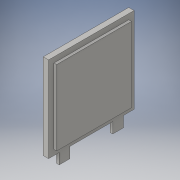
# Autodesk Inventor part: top
Saved by Autodesk Inventor 2016 (Build 200138000, 138)
## iProperties
Created: 2016-08-07
Part Number: top
Material: Generic
Document SubType Name: Modeling
Designer: Jorian Brusind
Density: 1 g/cm^3
Appearance: Default
Author: Jorian Brusind
Autodesk Inventor part; units mm, degrees
ref_plane "YZ Plane" through (0, 0, 0) normal (1, 0, 0) x (0, 1, 0)
ref_plane "XZ Plane" through (0, 0, 0) normal (0, 1, 0) x (-1, 0, 0)
ref_plane "XY Plane" through (0, 0, 0) normal (0, 0, 1) x (1, 0, 0)
sketch "Sketch1" plane through (0, 0, 0) normal (0, 1, 0) x (-1, 0, 0)
  line L0 (0, 0) -> (6.35, 0)
  line L1 (6.35, 0) -> (6.35, -101.6)
  line L2 (6.35, -101.6) -> (0, -101.6)
  line L3 (0, -101.6) -> (0, 0)
  dimension "d0" = 6.35
  dimension "d1" = 101.6
  constraints: 8 end point, 2 parallel, 1 horizontal, 1 perpendicular
  measures "d0" distance of L1.end L2.end
  measures "d1" distance of L0.end L1.end
extrude "Extrusion1" add sketch "Sketch1" along normal blind 101.6
sketch "Sketch2" plane through (0, 0, 0) normal (0, -1, 0) x (1, 0, 0)
  line L0 (0, 0) -> (0, -25.4)
  line L1 (0, 0) -> (0, -101.6) projected
  line L2 (0, -101.6) -> (0, -76.2)
  line L3 (0, -25.4) -> (-3.175, -25.4)
  line L4 (-3.175, -25.4) -> (-3.175, -12.7)
  line L5 (-3.175, -12.7) -> (0, -12.7)
  line L6 (0, -12.7) -> (0, -25.4)
  line L7 (0, -76.2) -> (-3.175, -76.2)
  line L8 (-3.175, -76.2) -> (-3.175, -88.9)
  line L9 (-3.175, -88.9) -> (0, -88.9)
  line L10 (0, -88.9) -> (0, -76.2)
  dimension "d4" = 25.4
  dimension "d5" = 25.4
  dimension "d6" = 3.175
  dimension "d7" = 12.7
  dimension "d8" = 3.175
  dimension "d9" = 12.7
  constraints: 20 end point, 4 parallel, 2 horizontal, 2 perpendicular, 2 point on line
  measures "d4" distance of L0.start L0.end
  measures "d5" distance of L1.end L2.end
  measures "d6" distance of L4.end L5.end
  measures "d7" distance of L3.end L4.end
  measures "d8" distance of L9.end L8.end
  measures "d9" distance of L8.end L7.end
extrude "Extrusion2" add sketch "Sketch2" along normal blind 12.7
sketch "Sketch3" plane through (0, 0, -101.6) normal (1, 0, 0) x (0, 0, -1)
  line L0 (0, 0) -> (0, 101.6) projected
  line L1 (0, 0) -> (-12.7, 0) projected
  line L2 (-101.6, 0) -> (-101.6, 101.6) projected
  line L3 (-95.25, 95.25) -> (-95.25, 6.35)
  line L4 (-95.25, 6.35) -> (-6.35, 6.35)
  line L5 (-6.35, 6.35) -> (-6.35, 95.25)
  line L6 (-6.35, 95.25) -> (-95.25, 95.25)
  line L7 (-101.6, 0) -> (0, 0) projected
  line L8 (0, 101.6) -> (-101.6, 101.6) projected
  dimension "d20" = 88.9
  dimension "d22" = 6.35
  dimension "d23" = 6.35
  dimension "d24" = 6.35
  constraints: 8 end point, 2 perpendicular, 1 horizontal
  measures "d20" distance of L3.end L4.end
  measures "d22" distance between parallel lines of L7 L4
  measures "d23" distance between parallel lines of L8 L6
  measures "d24" distance between parallel lines of L2 L3
extrude "Extrusion4" add sketch "Sketch3" along normal blind 3.175 contours L6 L5 L4 L3
body "Solid1"
